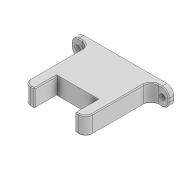
# Autodesk Inventor part: base_servo
Saved by Autodesk Inventor 2022 (Build 260153000, 153)
## iProperties
Created: 2022-11-06
Part Number: base_servo
Material: Genérico
Document SubType Name: Modeling
Designer: Jorge
Density: 1 g/cm^3
Appearance: Valor por defecto
Author: Jorge
Autodesk Inventor part; units mm, degrees
ref_plane "YZ Plane" through (0, 0, 0) normal (1, 0, 0) x (0, 1, 0)
ref_plane "XZ Plane" through (0, 0, 0) normal (0, 1, 0) x (-1, 0, 0)
ref_plane "XY Plane" through (0, 0, 0) normal (0, 0, 1) x (1, 0, 0)
sketch "Boceto1" plane through (0, 0, 0) normal (0, 0, 1) x (1, 0, 0)
  line L0 (0, 0) -> (35, 0)
  line L1 (35, 0) -> (35, 10)
  line L2 (35, 10) -> (0, 10)
  line L3 (0, 10) -> (0, 0)
  dimension "d0" = 35
  dimension "d1" = 10
  constraints: 8 end point, 2 parallel, 1 horizontal, 1 perpendicular
  measures "d0" distance of L2.end L1.end
  measures "d1" distance of L1.end L0.end
extrude "Extrusión1" add sketch "Boceto1" along normal blind 40
sketch "Boceto2" plane through (0, 0, 40) normal (0, 0, 1) x (1, 0, 0)
  line L0 (35, 0) -> (35, 10) construction
  line L1 (35, 10) -> (0, 10) construction
  line L2 (0, 10) -> (0, 0) construction
  line L3 (0, 0) -> (35, 0) construction
  line L4 (35, 10) -> (0, 10) projected
  line L5 (0, 0) -> (35, 0) projected
  line L6 (6, 10) -> (29, 10)
  line L7 (29, 10) -> (29, 0)
  line L8 (29, 0) -> (6, 0)
  line L9 (6, 0) -> (6, 10)
  line L10 (17.5, 10) -> (17.5, 0) construction
  dimension "d4" = 23
  dimension "d5" = 11.5
  constraints: 10 end point, 2 midpoint, 2 parallel, 2 point on line, 1 horizontal, 1 perpendicular
  measures "d4" distance of L7.end L8.end
  measures "d5" distance between parallel lines of L10 L9
extrude "Extrusión2" cut sketch "Boceto2" against normal blind 13
sketch "Boceto3" plane through (0, 0, 0) normal (0, 0, -1) x (-1, 0, 0)
  line L0 (-35, 0) -> (-35, 10) construction
  line L1 (0, 0) -> (-35, 0) construction
  line L2 (0, 10) -> (0, 0) construction
  line L3 (-35, 10) -> (0, 10) construction
  line L4 (-35, 10) -> (-45, 10)
  line L5 (-45, 10) -> (-45, 0)
  line L6 (-45, 0) -> (-35, 0)
  line L7 (-35, 0) -> (-35, 10)
  line L8 (-6, 10) -> (0, 10) projected
  line L9 (0, 10) -> (10, 10)
  line L10 (10, 10) -> (10, 0)
  line L11 (10, 0) -> (0, 0)
  line L12 (0, 0) -> (0, 10)
  line L13 (-35, 0) -> (-35, 10) construction
  line L14 (0, 10) -> (0, 0) construction
  dimension "d8" = 10
  dimension "d9" = 10
  constraints: 16 end point, 4 parallel, 2 horizontal, 2 perpendicular, 1 point on line
  measures "d8" distance of L6.end L5.end
  measures "d9" distance of L10.end L11.end
extrude "Extrusión3" add sketch "Boceto3" against normal blind 3
fillet "Empalme1" radius 4 8 edges at (-10, 0, 1.5) (-10, 10, 1.5) (45, 0, 1.5) (45, 10, 1.5) (0, 5, 40) (35, 5, 40) (0, 5, 3) (35, 5, 3)
sketch "Boceto5" plane through (0, 0, 3) normal (0, 0, 1) x (1, 0, 0)
  line L0 (-4, 10) -> (-4, 0) construction
  line L1 (-4, 10) -> (-6, 10) construction
  arc A0 (-6, 10) -> (-10, 6) centre (-6, 6) ccw construction
  line L2 (-10, 6) -> (-10, 4) construction
  arc A1 (-10, 4) -> (-6, 0) centre (-6, 4) ccw construction
  line L3 (-6, 0) -> (-4, 0) construction
  line L4 (39, 0) -> (39, 10) construction
  line L5 (39, 0) -> (41, 0) construction
  arc A2 (41, 0) -> (45, 4) centre (41, 4) ccw construction
  line L6 (45, 4) -> (45, 6) construction
  arc A3 (45, 6) -> (41, 10) centre (41, 6) ccw construction
  line L7 (41, 10) -> (39, 10) construction
  line L8 (-10, 5) -> (45, 5) construction
  circle A4 centre (-6.5, 5) radius 1.6
  circle A5 centre (41.5, 5) radius 1.6
  point P0 (0, 0)
  dimension "d15" = 3.2
  dimension "d16" = 3.2
  dimension "d17" = 3.5
  dimension "d18" = 3.5
  constraints: 2 centre point, 2 end point, 2 midpoint, 2 point on line
  measures "d15" diameter of A4
  measures "d16" diameter of A5
  measures "d17" distance from line of L6 A5.centre
  measures "d18" distance from line of L2 A4.centre
extrude "Extrusión4" cut sketch "Boceto5" against normal blind 10
chamfer "Chaflán1" distance 0.5 angle 45 28 edges at (-8.8284, 1.1716, 3) (-10, 5, 3) (-8.8284, 8.8284, 3) (-5, 10, 3) (0, 10, 21.5) (1.1716, 10, 38.8284) (5, 10, 40) (-5, 0, 3) (0, 0, 21.5) (1.1716, 0, 38.8284) (5, 0, 40) (40, 0, 3) (43.8284, 1.1716, 3) (45, 5, 3) (43.8284, 8.8284, 3) (40, 10, 3) (35, 10, 21.5) (33.8284, 10, 38.8284) (30, 10, 40) (35, 0, 21.5) (33.8284, 0, 38.8284) (30, 0, 40) (6, 5, 40) (29, 5, 40) (6, 0, 33.5) (6, 10, 33.5) (29, 0, 33.5) (29, 10, 33.5)
sketch "Boceto6" plane through (-6, 0, 0) normal (0, -1, 0) x (1, 0, 0)
  line L0 (45, 2.5) -> (47, 2.5) construction
  arc A0 (40.5, 7) -> (45, 2.5) centre (45, 7) ccw construction
  line L1 (40.5, 36) -> (40.5, 7) construction
  arc A1 (40.5, 36) -> (37, 39.5) centre (37, 36) ccw construction
  line L2 (35.5, 39.5) -> (37, 39.5) construction
  line L3 (35.5, 27) -> (35.5, 39.5) construction
  line L4 (35.5, 27) -> (11.5, 27) construction
  line L5 (11.5, 39.5) -> (11.5, 27) construction
  line L6 (10, 39.5) -> (11.5, 39.5) construction
  arc A2 (10, 39.5) -> (6.5, 36) centre (10, 36) ccw construction
  line L7 (6.5, 7) -> (6.5, 36) construction
  arc A3 (2, 2.5) -> (6.5, 7) centre (2, 7) ccw construction
  line L8 (0, 2.5) -> (2, 2.5) construction
  line L9 (0, 0) -> (0, 2.5) construction
  line L10 (47, 0) -> (0, 0) construction
  line L11 (47, 2.5) -> (47, 0) construction
  arc A4 (10, 39.5) -> (6.5, 36) centre (10, 36) ccw construction
  line L12 (9.5, 39.4641) -> (9.5, 0) construction
  line L13 (47, 0) -> (0, 0) construction
  arc A5 (40.5, 36) -> (37, 39.5) centre (37, 36) ccw construction
  line L14 (37.5, 39.4641) -> (37.5, 0) construction
  line L15 (23.5, 0) -> (23.5, 27) construction
  line L16 (6.5, 33.2) -> (40.5, 33.2) construction
  line L17 (40.5, 7) -> (40.5, 36) construction
  circle A6 centre (9.5, 33.2) radius 1.75
  circle A7 centre (37.5, 33.2) radius 1.75
  point P0 (6, 0)
  dimension "d26" = 28
  dimension "d27" = 14
  dimension "d28" = 6.2
  dimension "d29" = 3.5
  dimension "d30" = 3.5
  constraints: 8 end point, 8 point on line, 3 perpendicular, 2 centre point, 2 midpoint, 2 point on circle
  measures "d26" distance between parallel lines of L14 L12
  measures "d27" distance between parallel lines of L15 L12
  measures "d28" distance between parallel lines of L4 L16
  measures "d29" diameter of A6
  measures "d30" diameter of A7
extrude "Extrusión5" cut sketch "Boceto6" against normal blind 5
equation "\"d5\" = 0.5 * d4"
equation "\"d27\" = 0.5 * d26"
